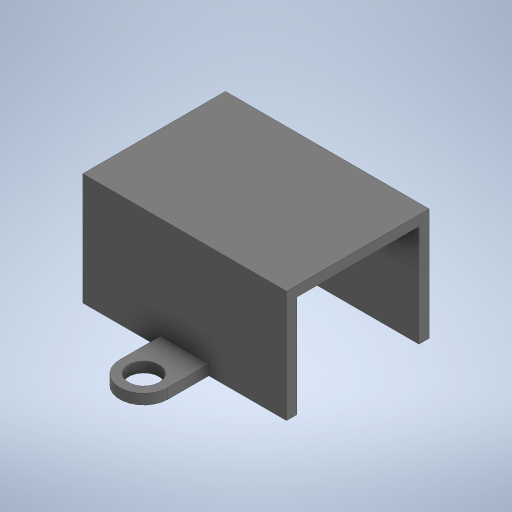
# Autodesk Inventor part: engate_motor
Saved by Autodesk Inventor 2023 (Build 270158000, 158)
## iProperties
Created: 2023-08-09
Part Number: engate_motor
Material: Genérico
Document SubType Name: Modeling
Designer: azeve
Density: 1 g/cm^3
Appearance: Padrão
Author: azeve
Autodesk Inventor part; units mm, degrees
ref_plane "YZ Plane" through (0, 0, 0) normal (1, 0, 0) x (0, 1, 0)
ref_plane "XZ Plane" through (0, 0, 0) normal (0, 1, 0) x (-1, 0, 0)
sketch "Esboço1" plane through (0, 0, 0) normal (1, 0, 0) x (0, 1, 0)
  line L0 (0, 0) -> (10, 0)
  line L1 (10, 1) -> (1, 1)
  line L2 (10, 0) -> (10, -12)
  line L3 (10, -12) -> (1, -12)
  line L4 (10, 1) -> (11, 1)
  line L5 (11, 1) -> (11, -13)
  line L6 (11, -13) -> (1, -13)
  line L7 (0, 1) -> (0, 0)
  line L8 (10, 0) -> (0, 0)
  line L9 (1, -12) -> (0, -12)
  line L10 (0, -12) -> (0, -13)
  line L11 (1, -13) -> (0, -13)
  line L12 (1, 1) -> (0, 1)
  constraints: 26 end point, 3 horizontal, 3 parallel, 3 vertical, 1 collinear, 1 perpendicular, 1 point on line
extrude "Extrusão1" add sketch "Esboço1" along normal blind 20
ref_plane "Plano de trabalho1" through (0, 0, 0) normal (0, -1, 0) x (1, 0, 0)
sketch "Esboço2" plane through (0, 0, 0) normal (0, -1, 0) x (1, 0, 0)
  line L0 (0, 0) -> (20, 0) projected
  line L1 (20, 0) -> (20, -12) projected
  line L2 (20, -6) -> (22.0296, -6)
  line L3 (0, 1) -> (20, 1) projected
  line L4 (10, 1) -> (10, 5.0127) construction
  line L5 (7.6336, 1) -> (7.6336, 5.0127)
  line L6 (12.3664, 5.0127) -> (12.3664, 1)
  arc A0 (12.3664, 5.0127) -> (7.6336, 5.0127) centre (10, 5.0127) ccw
  circle A1 centre (10, 5.0127) radius 1.5
  line L7 (7.6336, -13) -> (7.6336, -17.0127)
  line L8 (12.3664, -17.0127) -> (12.3664, -13)
  arc A2 (7.6336, -17.0127) -> (12.3664, -17.0127) centre (10, -17.0127) ccw
  circle A3 centre (10, -17.0127) radius 1.5
  line L9 (12.3664, -13) -> (7.6336, -13)
  line L10 (0, -13) -> (20, -13) projected
  line L11 (12.3664, 1) -> (7.6336, 1)
  point P0 (10, 3.0064)
  constraints: 18 end point, 6 symmetric about line, 4 centre point, 4 point on circle, 3 midpoint, 2 coincident, 2 perpendicular, 2 tangent, 1 collinear, 1 horizontal, 1 parallel, 2 other
extrude "Extrusão2" add sketch "Esboço2" against normal blind 1
